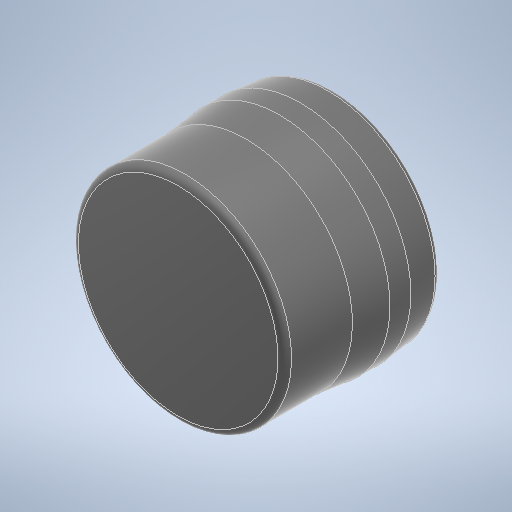
# Autodesk Inventor part: Spring_Top_2
Saved by Autodesk Inventor 2025.1 (Build 291241020, 241B)
## iProperties
Created: 2024-11-13
Part Number: Spring_Top_2
Material: PC/ABS Plastic
Document SubType Name: Modeling
Designer: leon-
Density: 1.1 g/cm^3
Appearance: Smooth - Black
Author: leon-
## iProperties of the stored document Spring_Top_3DPrint.ipt
Created: 2024-11-16
Part Number: Spring_Top_3DPrint
Material: Generic
Document SubType Name: Modeling
Designer: leon-
Density: 1 g/cm^3
Appearance: Default
Author: leon-
Autodesk Inventor part; units mm, degrees
ref_plane "YZ Plane" through (0, 0, 0) normal (1, 0, 0) x (0, 1, 0)
ref_plane "XZ Plane" through (0, 0, 0) normal (0, 1, 0) x (-1, 0, 0)
ref_plane "XY Plane" through (0, 0, 0) normal (0, 0, 1) x (1, 0, 0)
sketch "Sketch1" plane through (0, 0, 0) normal (1, 0, 0) x (0, 1, 0)
  line L0 (0, 0) -> (15.75, 0)
  line L1 (15.75, 0) -> (15.75, -10)
  line L2 (15.75, -10) -> (10.2, -10)
  line L3 (10.2, -10) -> (10.2, -5)
  line L4 (10.2, -5) -> (0, -5)
  line L5 (0, -5) -> (0, 0)
  point P0 (0, -2.5)
  point P1 (15.75, -5)
  point P2 (7.875, 0)
  dimension "d0" = 15.75
  dimension "d1" = 10.2
  dimension "d2" = 10
  dimension "d3" = 5
  constraints: 12 end point, 5 perpendicular, 3 midpoint, 1 horizontal
  measures "d0" horizontal distance of point (0, -2.5) point (15.75, -5)
  measures "d1" distance between parallel lines of L5 L3
  measures "d2" distance between parallel lines of L0 L2
  measures "d3" distance from line of point (7.875, 0) L4
revolve "Revolution1" add sketch "Sketch1" angle 360 about axis through (0, 0, -5) along (0, 0, 1)
sketch "Sketch3" plane through (0, 0, 0) normal (1, 0, 0) x (0, 1, 0)
  line L0 (15.75, 0) -> (-15.75, 0) projected
  line L1 (15.75, -10) -> (-15.75, -10) projected
  line L2 (15.75, -10) -> (15.75, 0) projected
  line L3 (15.75, -10) -> (16.3, -15)
  line L4 (15.5, -15.0439) -> (14.9452, -10)
  line L5 (14.9452, -10) -> (15.75, -10)
  line L6 (0, -24.0479) -> (0, 4.008) projected
  line L7 (16.3, -15) -> (16.3, -18.0877)
  line L8 (15.5, -18.0439) -> (15.5, -15.0439)
  line L9 (15.5, -18.0439) -> (14.9548, -23.0003)
  line L10 (14.9548, -23.0003) -> (15.75, -23.0877)
  line L11 (15.75, -23.0877) -> (16.3, -18.0877)
  point P0 (0, 0)
  point P1 (0, 0)
  point P2 (15.2274, -20.5221)
  dimension "d14" = 0.8
  dimension "d15" = 16.3
  dimension "d16" = 5
  dimension "d19" = 0.8
  dimension "d21" = 3
  dimension "d22" = 5
  dimension "d25" = 0.8
  constraints: 16 end point, 2 midpoint, 1 collinear, 1 parallel, 1 perpendicular, 1 vertical, 1 vertical alignment
  measures "d14" distance between parallel lines of L3 L4
  measures "d15" horizontal distance of point (0, 0) L3.end
  measures "d16" distance from line of L1 L3.end
  measures "d19" distance between parallel lines of L7 L8
  measures "d21" distance of L8.start L4.start
  measures "d22" vertical distance of L7.end L10.end
  measures "d25" distance between parallel lines of L9 L11
revolve "Revolution2" add sketch "Sketch3" angle 360 about axis through (0, 0, -10) along (0, 0, 1) contours L3 L7 L11 L10 L9 L8 L4 L1
fillet "Fillet2" radius 1 2 edges at (0, -15.75, 0) (0, -15.75, -23.0877)
body "Solid1"
